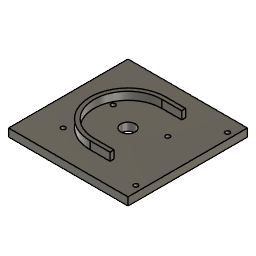
Pump Assembly (Autodesk Fusion 360 archive; units mm, degrees)
design "stepper motor base v1"
part number: 2026-04-22-00-17-38-220
Autodesk Fusion 360 part; units mm, degrees
sketch "Sketch1" plane through (0, 0, 0) normal (0, 1, 0) x (1, 0, 0)
  line L0 (38.1, 38.1) -> (-38.1, 38.1)
  line L1 (-38.1, 38.1) -> (-38.1, -38.1)
  line L2 (-38.1, -38.1) -> (38.1, -38.1)
  line L3 (38.1, -38.1) -> (38.1, 38.1)
  line L4 (38.1, 38.1) -> (-38.1, -38.1) construction
  line L5 (-38.1, 38.1) -> (38.1, -38.1) construction
  dimension "d1" = 76.2
  dimension "d2" = 76.2
  constraint horizontal L0
  constraint perpendicular L0 L1
  constraint parallel L0 L2
  constraint parallel L1 L3
  constraint coincident L4 origin
  constraint coincident L5 origin
  measures "d1" distance of L1.end L2.end
  measures "d2" distance of L0.end L1.end
extrude "Extrude1" add sketch "Sketch1" along normal blind 5.08
sketch "Sketch2" plane through (0, 5.08, 0) normal (0, 1, 0) x (-1, 0, 0)
  line L0 (-38.1, 38.1) -> (-38.1, -38.1)
  line L1 (-38.1, -38.1) -> (38.1, -38.1)
  line L2 (38.1, -38.1) -> (38.1, 38.1)
  line L3 (38.1, 38.1) -> (-38.1, 38.1)
  circle A0 centre (-17.399, -8) radius 1.4
  circle A1 centre (17.399, -8) radius 1.4
  line L4 (0, 1.75) -> (0, 22.5)
  circle A2 centre (0, 0) radius 4.572
  line L5 (-50.0726, -8) -> (46.4474, -8) construction
  dimension "d5" = 34.798
  dimension "d6" = 2.8
  dimension "d7" = 2.8
  dimension "d8" = 9.144
  dimension "d9" = 8
  constraint symmetric A0.centre A1.centre L4
  constraint coincident L4 A2.centre
  constraint horizontal L5
  constraint coincident A2.centre origin
  constraint coincident A0.centre L5
  measures "d5" distance of A0.centre A1.centre
  measures "d6" diameter of A0
  measures "d7" diameter of A1
  measures "d8" diameter of A2
  measures "d9" distance of A2.centre L5
extrude "Extrude2" cut sketch "Sketch2" against normal through all contours A0 | A1 | A2
sketch "Sketch3" plane through (0, 5.08, 0) normal (0, 1, 0) x (-1, 0, 0)
  circle A0 centre (0, 0) radius 4.572
  circle A1 centre (-17.399, -8) radius 1.4
  circle A2 centre (17.399, -8) radius 1.4
  line L0 (-38.1, 38.1) -> (-38.1, -38.1)
  line L1 (-38.1, -38.1) -> (38.1, -38.1)
  line L2 (38.1, -38.1) -> (38.1, 38.1)
  line L3 (38.1, 38.1) -> (-38.1, 38.1)
  line L4 (0, 44.3572) -> (0, -39.4628) construction
  line L5 (0, 1.75) -> (0, 22.5)
  arc A3 (0, -21.59) -> (0, 21.59) centre (0, 0) ccw
  arc A4 (0, -24.13) -> (0, 24.13) centre (0, 0) ccw
  line L6 (0, 24.13) -> (-12.7, 24.13)
  line L7 (-12.7, 24.13) -> (-12.7, 21.59)
  line L8 (-12.7, 21.59) -> (0, 21.59)
  line L9 (0, -21.59) -> (-12.7, -21.59)
  line L10 (-12.7, -21.59) -> (-12.7, -24.13)
  line L11 (-12.7, -24.13) -> (0, -24.13)
  dimension "d11" = 43.18
  dimension "d12" = 48.26
  dimension "d13" = 12.7
  dimension "d14" = 12.7
  constraint concentric A0 A3
  constraint concentric A3 A4
  constraint parallel L0 L4
  constraint collinear L4 L5
  constraint coincident L4 A3.end
  constraint coincident L4 A3.start
  constraint coincident L4 A4.end
  constraint coincident L4 A4.start
  constraint tangent A4 L6
  constraint perpendicular L6 L7
  constraint tangent A3 L8
  constraint tangent A3 L9
  constraint perpendicular L9 L10
  constraint tangent A4 L11
  measures "d11" diameter of A3
  measures "d12" diameter of A4
  measures "d13" distance of L4 L7
  measures "d14" distance of L4 L10
extrude "Extrude3" add sketch "Sketch3" along normal blind 5 contours A3 A4 L6 L7 L8 L9 L10 L11
sketch "Sketch4" plane through (0, 5.08, 0) normal (0, 1, 0) x (-1, 0, 0)
  arc A0 (0, -21.59) -> (0, 21.59) centre (0, 0) ccw
  line L0 (0, 21.59) -> (-12.7, 21.59)
  line L1 (-12.7, 21.59) -> (-12.7, 24.13)
  line L2 (-12.7, 24.13) -> (0, 24.13)
  arc A1 (0, -24.13) -> (0, 24.13) centre (0, 0) ccw
  line L3 (0, -24.13) -> (-12.7, -24.13)
  line L4 (-12.7, -24.13) -> (-12.7, -21.59)
  line L5 (-12.7, -21.59) -> (0, -21.59)
  circle A2 centre (0, 0) radius 4.572
  circle A3 centre (-17.399, -8) radius 1.4
  circle A4 centre (17.399, -8) radius 1.4
  line L6 (-38.1, 38.1) -> (-38.1, -38.1)
  line L7 (-38.1, -38.1) -> (38.1, -38.1)
  line L8 (38.1, -38.1) -> (38.1, 38.1)
  line L9 (38.1, 38.1) -> (-38.1, 38.1)
  circle A5 centre (-34.29, 29.21) radius 1.4
  circle A6 centre (20.6553, 20.6553) radius 1.4
  dimension "d17" = 2.8
  dimension "d18" = 2.8
  dimension "d21" = 3.81
  dimension "d22" = 8.89
  dimension "d26" = 17.4447
  dimension "d27" = 17.4447
  measures "d17" diameter of A5
  measures "d18" diameter of A6
  measures "d21" distance of L6 A5.centre
  measures "d22" distance of L9 A5.centre
  measures "d26" distance of L9 A6.centre
  measures "d27" distance of L8 A6.centre
extrude "Extrude4" cut sketch "Sketch4" against normal through all contours A5 | A6
mirror "Mirror1" about plane through (0, 0, 0) normal (0, 0, 1) of "Extrude4"
move_body "Move1" bodies 1 to x (1, 0, 0) y (0, 0, 1) z (0, -1, 0) at (0, 15.2757, 5.1157)

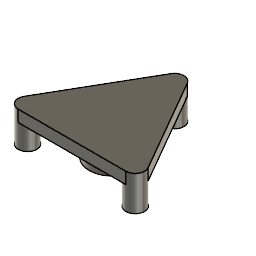
design "bearing rotor v1"
part number: 2026-04-22-23-42-39-207
Autodesk Fusion 360 part; units mm, degrees
sketch "Sketch1" plane through (0, 0, 0) normal (0, 0, 1) x (1, 0, 0)
  circle A0 centre (0, 0) radius 21.59 construction
  line L0 (0, 27.546) -> (0, -31.973) construction
  line L1 (-40.4824, 0) -> (36.5438, 0) construction
  line L2 (0, 1.75) -> (0, 22.5)
  line L3 (1.75, 0) -> (22.5, 0)
  line L4 (-2, 1.5) -> (2, 1.5)
  line L5 (-2, -1.5) -> (2, -1.5)
  circle A1 centre (0, 0) radius 5.08
  arc A2 (-2, 1.5) -> (-2, -1.5) centre (0, 0) ccw
  arc A3 (2, -1.5) -> (2, 1.5) centre (0, 0) ccw
  circle A4 centre (0, 13.566) radius 6.5 construction
  circle A5 centre (0, 13.566) radius 2.05
  line L6 (7.62, 20.066) -> (-7.158, 20.066) construction
  line L7 (-11.43, 21.59) -> (19.6746, 21.59) construction
  dimension "d1" = 43.18
  dimension "d3" = 5
  dimension "d4" = 3
  dimension "d5" = 10.16
  dimension "d6" = 2.5
  dimension "d7" = 13
  dimension "d8" = 4.1
  dimension "d18" = 1.524
  constraint coincident A0.centre A1.centre
  constraint vertical L0
  constraint horizontal L1
  constraint collinear L0 L2
  constraint collinear L1 L3
  constraint concentric A0 A2
  constraint perpendicular L0 L4
  constraint perpendicular L0 L5
  constraint symmetric L1 L4 L5
  constraint concentric A0 A1
  constraint concentric A2 A3
  constraint coincident L0 A4.centre
  constraint concentric A4 A5
  constraint horizontal L6
  constraint horizontal L7
  constraint tangent A4 L6
  constraint tangent A0 L7
  measures "d1" diameter of A0
  measures "d3" diameter of A2
  measures "d4" distance of L4 L5
  measures "d5" diameter of A1
  measures "d6" radius of A3
  measures "d7" diameter of A4
  measures "d8" diameter of A5
  measures "d18" distance of L6 L7
extrude "Extrude1" add sketch "Sketch1" along normal blind 5.08 makes body 1 at (2.0398, 13.3619, 1.6933) makes body 2 at (5.0548, -0.5058, 1.6933)
pattern_circular "C-Pattern4" count 3 over 360 about axis through (0, 0, 1.75) along (0, 0, 1) of bodies 1 makes body 3 at (-12.5916, -4.9144, 1.6933) makes body 4 at (10.5518, -8.4475, 1.6933)
sketch "Sketch3" plane through (0, 0, 5.08) normal (0, 0, 1) x (-1, 0, 0)
  arc A0 (2, -1.5) -> (2, 1.5) centre (0, 0) ccw
  line L0 (2, -1.5) -> (-2, -1.5)
  arc A1 (-2, 1.5) -> (-2, -1.5) centre (0, 0) ccw
  line L1 (-2, 1.5) -> (2, 1.5)
  circle A2 centre (0, 0) radius 5.08
  line L2 (13.5239, 5.758) -> (1.7754, -14.591)
  line L3 (-1.7754, -14.591) -> (-13.5239, 5.758)
  line L4 (11.7485, 8.833) -> (-11.7485, 8.833)
  circle A3 centre (11.7485, 6.783) radius 2.05
  circle A4 centre (0, -13.566) radius 2.05
  circle A5 centre (-11.7485, 6.783) radius 2.05
  constraint horizontal L4
  constraint coincident L2.start A3
  constraint coincident L2.end A4
  constraint coincident L3.start A4
  constraint coincident L3.end A5
  constraint coincident L4.end A5
  constraint coincident L4.start A3
  constraint tangent L3 A4
  constraint tangent L2 A4
  constraint tangent L3 A5
  constraint tangent L2 A3
  constraint tangent L4 A3
extrude "Extrude4" add sketch "Sketch3" along normal blind 2.54 contours A0 L0 A1 L1 | A2 | L2 L3 L4 A3 A4 A5 | A3 | A4 | A5 bodies 1 2 3 4

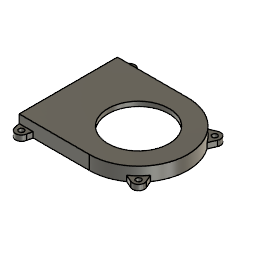
design "Rotor Housing"
part number: 2026-05-21-21-26-19-566
Autodesk Fusion 360 part; units mm, degrees
sketch "Sketch1" plane through (0, 0, 0) normal (0, 0, 1) x (1, 0, 0)
  line L0 (0, 26.67) -> (-38.1, 26.67)
  line L1 (0, -26.67) -> (-38.1, -26.67)
  line L2 (-38.1, 24.257) -> (0, 24.257)
  line L3 (-38.1, -24.257) -> (0, -24.257)
  line L4 (-38.1, 26.67) -> (-38.1, 24.257)
  line L5 (-38.1, -24.257) -> (-38.1, -26.67)
  arc A0 (0, -26.67) -> (0, 26.67) centre (0, 0) ccw
  arc A1 (0, -24.257) -> (0, 24.257) centre (0, 0) ccw
  dimension "d1" = 53.34
  dimension "d2" = 48.514
  dimension "d3" = 38.1
  dimension "d4" = 38.1
  constraint coincident A0.centre A1.centre
  constraint horizontal L0
  constraint horizontal L1
  constraint tangent L0 A0
  constraint tangent L1 A0
  constraint horizontal L2
  constraint parallel L1 L3
  constraint tangent L2 A1
  constraint tangent L3 A1
  constraint vertical L4
  constraint perpendicular L1 L5
  constraint coincident L0.end L4.start
  constraint coincident L2.start L4.end
  constraint coincident L3.start L5.start
  constraint coincident L1.end L5.end
  measures "d1" diameter of A0
  measures "d2" diameter of A1
  measures "d3" distance of L0.start L0.end
  measures "d4" distance of L1.start L1.end
extrude "Extrude1" add sketch "Sketch1" along normal blind 5
sketch "Sketch2" plane through (0, 0, 5) normal (0, 0, 1) x (-1, 0, 0)
  line L0 (38.1, 24.257) -> (38.1, 26.67)
  line L1 (38.1, 26.67) -> (0, 26.67)
  arc A0 (0, 26.67) -> (0, -26.67) centre (0, 0) ccw
  line L2 (0, -26.67) -> (38.1, -26.67)
  line L3 (38.1, -26.67) -> (38.1, -24.257)
  line L4 (38.1, -24.257) -> (0, -24.257)
  arc A1 (0, 24.257) -> (0, -24.257) centre (0, 0) ccw
  line L5 (0, 24.257) -> (38.1, 24.257)
  line L6 (38.1, -26.67) -> (38.1, 26.67)
  constraint coincident L2.end L3.start
  constraint coincident L0.end L1.start
extrude "Extrude2" add sketch "Sketch2" along normal blind 2.54
sketch "Sketch3" plane through (0, 0, 7.54) normal (0, 0, 1) x (-1, 0, 0)
  line L0 (38.1, -26.67) -> (38.1, 26.67)
  line L1 (38.1, 26.67) -> (0, 26.67)
  arc A0 (0, 26.67) -> (0, -26.67) centre (0, 0) ccw
  line L2 (0, -26.67) -> (38.1, -26.67)
  circle A1 centre (0, 0) radius 16.51
  dimension "d9" = 33.02
  constraint concentric A0 A1
  measures "d9" diameter of A1
extrude "Extrude3" cut sketch "Sketch3" against normal through all contours A1
sketch "Sketch4" plane through (0, 0, 5) normal (0, 0, -1) x (1, 0, 0)
  circle A0 centre (0, 0) radius 16.51
  line L0 (0, 24.257) -> (-38.1, 24.257)
  line L1 (-38.1, 24.257) -> (-38.1, -24.257)
  line L2 (-38.1, -24.257) -> (0, -24.257)
  arc A1 (0, -24.257) -> (0, 24.257) centre (0, 0) ccw
  line L3 (-38.1, 19.257) -> (-35.56, 19.257)
  line L4 (-35.56, 19.257) -> (-35.56, -19.257)
  line L5 (-35.56, -19.257) -> (-38.1, -19.257)
  line L6 (-38.1, -19.257) -> (-38.1, 19.257)
  dimension "d11" = 5
  dimension "d12" = 5
  constraint horizontal L3
  constraint vertical L4
  constraint horizontal L5
  constraint vertical L6
  constraint coincident L1 L3.start
  measures "d11" distance of L0 L3
  measures "d12" distance of L2 L5
extrude "Extrude4" add sketch "Sketch4" along normal blind 5 contours L1 L3 L4 L5 L6
sketch "Sketch5" plane through (0, 0, 0) normal (0, 0, 1) x (1, 0, 0)
  line L0 (0, 0) -> (30.48, 30.48) construction
  line L1 (0, 0) -> (43.1052, 0) construction
  line L2 (0, 0) -> (33.4313, -33.4313) construction
  line L3 (0, 0) -> (47.279, 0) construction
  circle A0 centre (20.6546, 20.6546) radius 1.4
  circle A1 centre (20.6546, -20.6546) radius 1.4
  circle A2 centre (20.6546, 20.6546) radius 3.175
  line L4 (19.3121, 23.5318) -> (15.3534, 21.8074)
  line L5 (23.5318, 19.3121) -> (21.8074, 15.3534)
  arc A3 (0, -26.67) -> (0, 26.67) centre (0, 0) ccw
  dimension "d15" = 45
  dimension "d16" = 45
  dimension "d17" = 2.8
  dimension "d18" = 2.8
  dimension "d19" = 29.21
  dimension "d20" = 29.21
  dimension "d21" = 6.35
  dimension "d22" = 4.318
  constraint horizontal L1
  constraint coincident L0.start L1.start
  constraint horizontal L3
  constraint coincident L0 A0.centre
  constraint coincident L2 A1.centre
  constraint concentric A0 A2
  constraint coincident A2 L4.start
  constraint coincident A2 L5.start
  constraint coincident L4.end A3
  constraint coincident L5.end A3
  constraint symmetric L0 L4 L5
  measures "d15" angle of L0 L1
  measures "d16" angle of L2 L3
  measures "d17" diameter of A1
  measures "d18" diameter of A0
  measures "d19" distance of L0.start A1.centre
  measures "d20" distance of L0.start A0.centre
  measures "d21" diameter of A2
  measures "d22" distance of L4.start L4.end
extrude "Extrude5" add sketch "Sketch5" along normal blind 3 contours A2 A3 | A2 L4 A3 | A2 L5 A3 picked at (18.4077, 19.9432)
mirror "Mirror1" about plane through (0, 0, 0) normal (0, 1, 0) of "Extrude5"
sketch "Sketch6" plane through (0, 0, 0) normal (0, 0, 1) x (1, 0, 0)
  circle A0 centre (-34.29, -29.21) radius 1.4
  line L0 (-38.1, 26.67) -> (-38.1, -26.67)
  line L1 (-38.1, -26.67) -> (0, -26.67)
  circle A1 centre (-34.29, -29.21) radius 3.175
  line L2 (-37.444, -29.5746) -> (-38.1, -26.67)
  line L3 (-31.136, -29.5746) -> (-30.48, -26.67)
  dimension "d27" = 2.8
  dimension "d28" = 3.81
  dimension "d29" = 2.54
  dimension "d30" = 6.35
  constraint concentric A0 A1
  constraint coincident A1 L2.start
  constraint coincident L0.end L1.start
  constraint coincident A1 L3.start
  constraint coincident L1 L3.end
  measures "d27" diameter of A0
  measures "d28" distance of A0.centre L0
  measures "d29" distance of A0.centre L1
  measures "d30" diameter of A1
extrude "Extrude6" add sketch "Sketch6" along normal blind 3 contours L1 A1 L2 | L1 A1 | L1 A1 L3 picked at (-34.3249, -27.0513)
mirror "Mirror2" about plane through (0, 0, 0) normal (0, 1, 0) of "Extrude6"
sketch "Sketch7" plane through (0, 0, 0) normal (0, 0, 1) x (1, 0, 0)
  line L0 (38.1, -38.1) -> (-38.1, -38.1) construction
  line L1 (-38.1, -38.1) -> (-38.1, 38.1) construction
  line L2 (-38.1, 38.1) -> (38.1, 38.1) construction
  line L3 (38.1, 38.1) -> (38.1, -38.1) construction
  line L4 (38.1, -38.1) -> (-38.1, 38.1) construction
  line L5 (-38.1, -38.1) -> (38.1, 38.1) construction
  dimension "d35" = 76.2
  dimension "d36" = 76.2
  constraint horizontal L0
  constraint perpendicular L0 L1
  constraint parallel L0 L2
  constraint parallel L1 L3
  constraint coincident L4 origin
  constraint coincident L5 origin
  measures "d35" distance of L1.end L2.end
  measures "d36" distance of L0.end L1.end
